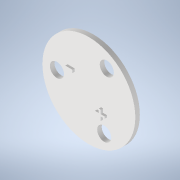
# Autodesk Inventor part: akkufach_deckel
Saved by Autodesk Inventor 2020.2 (Build 242310000, 310)
## iProperties
Created: 2020-11-08
Part Number: akkufach_deckel
Material: Generisch
Document SubType Name: Modeling
Designer: g.schardt
Density: 1 g/cm^3
Appearance: Vorgabe
Author: g.schardt
Autodesk Inventor part; units mm, degrees
ref_plane "YZ Plane" through (0, 0, 0) normal (1, 0, 0) x (0, 1, 0)
ref_plane "XZ Plane" through (0, 0, 0) normal (0, 1, 0) x (-1, 0, 0)
ref_plane "XY Plane" through (0, 0, 0) normal (0, 0, 1) x (1, 0, 0)
sketch "Skizze1" plane through (0, 0, 0) normal (0, 0, 1) x (1, 0, 0)
  circle A0 centre (0, 0) radius 20.4
  dimension "d0" = 40.8
  constraints: 1 centre point, 1 coincident
  measures "d0" diameter of A0
extrude "Extrusion1" add sketch "Skizze1" against normal blind 2
sketch "Skizze2" plane through (0, 0, 0) normal (0, 0, 1) x (1, 0, 0)
  circle A0 centre (10.4908, -0.4387) radius 8.6464 projected
  circle A1 centre (-5.6254, -8.866) radius 9 projected
  circle A2 centre (-4.8655, 9.3047) radius 8.6464 projected
  circle A3 centre (0, 0) radius 20.5 projected
  circle A4 centre (-14.0161, 0.868) radius 3.1
  line L0 (-4.8655, 0.6582) -> (-4.8655, 0.1019) construction
  line L1 (-20.4642, 1.2118) -> (10.4908, -0.4387) construction
  circle A5 centre (6.2563, -12.5723) radius 3.1
  circle A6 centre (7.7598, 11.7043) radius 3.1
  point P0 (0, 0)
  point P1 (6.7426, -12.9951)
  point P2 (7.8827, 12.3368)
  dimension "d15" = 6.2
  dimension "d22" = 360
  constraints: 4 end point, 3 centre point, 1 point on line, 1 vertical, 1 vertical alignment, 12 other
  measures "d15" diameter of A4
hole "Bohrung1" at (6.7426, -12.9951, 0) at (-14.0161, 0.868, 0) at (7.8827, 12.3368, 0) direction (0, 0, -1) diameter 6.2 end through all
sketch "Skizze3" plane through (0, 0, 0) normal (0, 0, 1) x (1, 0, 0)
  line L0 (2.9844, -3.6305) -> (8.6125, -3.6305) construction
  line L1 (8.6125, -3.6305) -> (8.6125, -10.4322) construction
  line L2 (8.6125, -10.4322) -> (2.9844, -10.4322) construction
  line L3 (2.9844, -10.4322) -> (2.9844, -3.6305) construction
  line L4 (-9.8763, 5.3535) -> (-5.1258, 5.3535) construction
  line L5 (-5.1258, 5.3535) -> (-5.1258, 3.2524) construction
  line L6 (-5.1258, 3.2524) -> (-9.8763, 3.2524) construction
  line L7 (-9.8763, 3.2524) -> (-9.8763, 5.3535) construction
  line L8 (7.9601, -6.2035) -> (6.2421, -6.2035)
  line L9 (6.2421, -6.2035) -> (6.2421, -7.9093)
  line L10 (6.2421, -7.9093) -> (5.3548, -7.9093)
  line L11 (5.3548, -7.9093) -> (5.3548, -6.2035)
  line L12 (5.3548, -6.2035) -> (3.6368, -6.2035)
  line L13 (3.6368, -6.2035) -> (3.6368, -5.3364)
  line L14 (3.6368, -5.3364) -> (5.3548, -5.3364)
  line L15 (5.3548, -5.3364) -> (5.3548, -3.6305)
  line L16 (5.3548, -3.6305) -> (6.2421, -3.6305)
  line L17 (6.2421, -3.6305) -> (6.2421, -5.3364)
  line L18 (6.2421, -5.3364) -> (7.9601, -5.3364)
  line L19 (7.9601, -5.3364) -> (7.9601, -6.2035)
  line L20 (-6.2458, 4.0488) -> (-9.3601, 4.0488)
  line L21 (-9.3601, 4.0488) -> (-9.3601, 5.3535)
  line L22 (-9.3601, 5.3535) -> (-6.2458, 5.3535)
  line L23 (-6.2458, 5.3535) -> (-6.2458, 4.0488)
  point P0 (0, 0)
  constraints: 4 other
extrude "Extrusion2" add sketch "Skizze3" along normal blind 1
